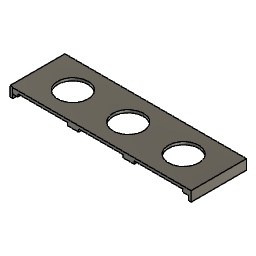
Storage_3DPrinting (Autodesk Fusion 360 design; units mm, degrees)
Autodesk Fusion 360 part; units mm, degrees
sketch "Sketch1" plane through (0, 0, 0) normal (0, 0, 1) x (1, 0, 0)
  line L0 (0, 0) -> (318, 0)
  line L1 (318, 0) -> (318, 100)
  line L2 (318, 100) -> (0, 100)
  line L3 (0, 100) -> (0, 0)
  line L4 (0, 100) -> (-5, 100)
  line L5 (-5, 100) -> (-5, 0.9365)
  line L6 (-5, 0.9365) -> (0, 0.9365)
  line L7 (0, 0.9365) -> (0, 100)
  line L8 (318, 100) -> (323, 100)
  line L9 (323, 100) -> (323, 0)
  line L10 (323, 0) -> (318, 0)
  line L11 (318, 0) -> (318, 100)
  line L12 (0, 50.4682) -> (318, 50.4682)
  circle A0 centre (159, 50.4682) radius 27.5
  line L13 (159, 50.4682) -> (59, 50.4682)
  circle A1 centre (59, 50.4682) radius 27.5
  line L14 (159, 50.4682) -> (259, 50.4682)
  circle A2 centre (259, 50.4682) radius 27.5
  line L15 (0, 100) -> (10, 100)
  line L16 (10, 100) -> (10, 0)
  line L17 (10, 0) -> (0, 0)
  line L18 (0, 0) -> (0, 100)
  line L19 (318, 100) -> (308, 100)
  line L20 (308, 100) -> (308, 0)
  line L21 (308, 0) -> (318, 0)
  line L22 (318, 0) -> (318, 100)
  line L23 (100, 100) -> (120, 100)
  line L24 (120, 100) -> (120, 0)
  line L25 (120, 0) -> (100, 0)
  line L26 (100, 0) -> (100, 100)
  line L27 (200, 100) -> (220, 100)
  line L28 (220, 100) -> (220, 0)
  line L29 (220, 0) -> (200, 0)
  line L30 (200, 0) -> (200, 100)
  dimension "d1" = 318
  dimension "d2" = 100
  dimension "d3" = 5
  dimension "d4" = 5
  dimension "d5" = 55
  dimension "d6" = 100
  dimension "d7" = 55
  dimension "d8" = 100
  dimension "d9" = 55
  dimension "d10" = 10
  constraint horizontal L0
  constraint vertical L1
  constraint horizontal L2
  constraint vertical L3
  constraint coincident L0.start L3.end
  constraint horizontal L4
  constraint vertical L5
  constraint horizontal L6
  constraint vertical L7
  constraint horizontal L8
  constraint vertical L9
  constraint horizontal L10
  constraint vertical L11
  constraint midpoint L7 L12.start
  constraint coincident L11 L12.end
  constraint perpendicular L11 L12
  constraint midpoint L12 A0.centre
  constraint coincident A0.centre L13.start
  constraint parallel L12 L13
  constraint coincident L13.end A1.centre
  constraint parallel L12 L14
  constraint coincident L14.end A2.centre
  constraint horizontal L15
  constraint vertical L16
  constraint horizontal L17
  constraint vertical L18
  constraint horizontal L19
  constraint vertical L20
  constraint horizontal L21
  constraint vertical L22
  constraint coincident L0 L20.end
  constraint horizontal L23
  constraint vertical L24
  constraint horizontal L25
  constraint vertical L26
  constraint coincident L0 L24.end
  constraint horizontal L27
  constraint vertical L28
  constraint horizontal L29
  constraint vertical L30
  constraint coincident L0 L28.end
  constraint coincident L2 L27.start
  measures "d1" distance of L0.start L0.end
  measures "d2" distance of L0.start L2.end
  measures "d3" distance of L2.end L4.end
  measures "d4" distance of L1.end L8.end
  measures "d5" diameter of A0
  measures "d6" distance of A0.centre L13.end
  measures "d7" diameter of A1
  measures "d8" distance of A0.centre L14.end
  measures "d9" diameter of A2
  measures "d10" distance of L1.end L19.end
extrude "Extrude1" add sketch "Sketch1" against normal blind 13 contours L3 L4 L5 L6 L7 L18 | L1 L8 L9 L10 L11 L22 makes body 1 at (-5, 66.9788, -4.3333) makes body 2 at (318, 33.3333, -8.6667)
extrude "Extrude2" add sketch "Sketch1" against normal blind 5 contours L0 L3 L7 L12 L16 L17 L18 | L0 L12 L13 L24 L25 L26 | L2 L3 L7 L12 L15 L16 L18 | L2 L12 L13 L23 L24 L26 | L0 L12 L14 L28 L29 L30 | L2 L12 L14 L27 L28 L30 | L0 L1 L11 L12 L20 L21 L22 | L1 L2 L11 L12 L19 L20 L22 bodies 1 2 makes body 3 at (106.6667, 66.6667, 0) makes body 4 at (206.6667, 66.6667, 0)
extrude "Extrude3" add sketch "Sketch1" along normal blind 5 contours L0 L3 L7 L12 L16 L17 L18 | L0 L12 L13 A1 L16 L26 | L3 L4 L5 L6 L7 L18 | L0 L12 L13 L24 L25 L26 | L2 L12 L13 A1 L16 L26 | L2 L3 L7 L12 L15 L16 L18 | L0 L12 A0 L13 L14 L24 L30 | L2 L12 L13 L23 L24 L26 | L0 L12 L14 L28 L29 L30 | L2 L12 A0 L13 L14 L24 L30 | L0 L12 L14 A2 L20 L28 | L2 L12 L14 L27 L28 L30 | L0 L1 L11 L12 L20 L21 L22 | L2 L12 L14 A2 L20 L28 | L1 L8 L9 L10 L11 L22 | L1 L2 L11 L12 L19 L20 L22 bodies 1 2 3 4
